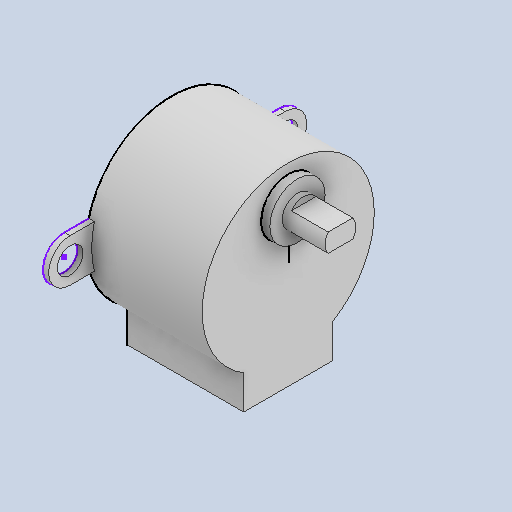
# Autodesk Inventor part: motor
Saved by Autodesk Inventor 2023 (Build 270158000, 158)
## iProperties
Created: 2022-04-18
Part Number: motor
Material: Generic
Document SubType Name: Modeling
Designer: carson
Density: 1 g/cm^3
Appearance: Default
Author: carson
Autodesk Inventor part; units mm, degrees
ref_plane "YZ Plane" through (0, 0, 0) normal (1, 0, 0) x (0, 1, 0)
ref_plane "XZ Plane" through (0, 0, 0) normal (0, 1, 0) x (-1, 0, 0)
ref_plane "XY Plane" through (0, 0, 0) normal (0, 0, 1) x (1, 0, 0)
sketch "Sketch1" plane through (0, 0, 0) normal (1, 0, 0) x (0, 1, 0)
  circle A0 centre (0, 0) radius 14
  line L0 (-6.3479, 7.25) -> (-17.5, 7.25)
  line L1 (-17.5, 7.25) -> (-17.5, -7.25)
  line L2 (-17.5, -7.25) -> (-6.3479, -7.25)
  circle A1 centre (-0.0001, 17.5) radius 3.5
  circle A2 centre (-0.0001, 17.5) radius 2.1
  line L3 (3.4999, 17.5) -> (3.4999, 13.5555)
  line L4 (-3.5001, 17.5) -> (-3.4999, 13.5555)
  line L5 (-14, 0) -> (14, 0)
  circle A3 centre (-0.0001, -17.5) radius 3.5
  circle A4 centre (-0.0001, -17.5) radius 2.1
  line L6 (3.4999, -17.5) -> (3.4999, -13.5555)
  line L7 (-3.5001, -17.5) -> (-3.4999, -13.5555)
  point P0 (-11.9765, -7.25)
  point P1 (-11.9765, 7.25)
  dimension "d0" = 28
  dimension "d7" = 14.5
  dimension "d8" = 7.25
  dimension "d9" = 17.5
  dimension "d12" = 7
  dimension "d13" = 4.2
  dimension "d14" = 17.5
  constraints: 16 end point, 8 point on circle, 6 symmetric about line, 5 centre point, 3 coincident, 2 horizontal, 1 parallel, 1 perpendicular, 1 tangent, 1 vertical, 2 other
  measures "d0" diameter of A0
  measures "d7" distance between parallel lines of L2 L0
  measures "d8" distance from line of A0.centre L2
  measures "d9" distance from line of A0.centre L1
  measures "d12" diameter of A1
  measures "d13" diameter of A2
  measures "d14" distance of point (0, 0) A2.centre
extrude "Extrusion1" add sketch "Sketch1" along normal blind 19 contours L5 A0 | A0 L5 | A0 L2 L1 L0
extrude "Extrusion2" add sketch "Sketch1" along normal blind 1 contours A0 A1 L3 | L6 A3 A0 | A0 L4 A1 | A1 | A3 L7 A0 | A3
sketch "Sketch3" plane through (19, 0, 0) normal (1, 0, 0) x (0, 0, -1)
  line L0 (0, 0) -> (0, 8)
  circle A0 centre (0, 8) radius 4.5
  circle A1 centre (0, 8) radius 2.5
  dimension "d17" = 8
  dimension "d18" = 9
  dimension "d19" = 5
  constraints: 2 centre point, 2 coincident, 2 end point, 1 vertical
  measures "d17" distance of L0.start L0.end
  measures "d18" diameter of A0
  measures "d19" diameter of A1
extrude "Extrusion3" add sketch "Sketch3" along normal blind 1.5
extrude "Extrusion4" add sketch "Sketch3" along normal blind 2.5 contours A1
sketch "Sketch5" plane through (21.5, 8, 0) normal (1, 0, 0) x (0, 0, -1)
  circle A0 centre (0, 0) radius 2.5 projected
  line L0 (-2, 1.5) -> (2, 1.5)
  circle A1 centre (0, 0) radius 2.5 projected
  line L1 (-2.5, 0) -> (2.5, 0)
  line L2 (-2, -1.5) -> (2, -1.5)
  point P0 (0, -8)
  dimension "d24" = 1.5
  constraints: 6 end point, 3 point on circle, 2 horizontal, 2 symmetric about line, 2 other
  measures "d24" distance from line of L0 point (0, 0)
extrude "Extrusion5" add sketch "Sketch5" along normal blind 6 contours L1 A0 L0 | A0 L2 L1
body "Solid1"
